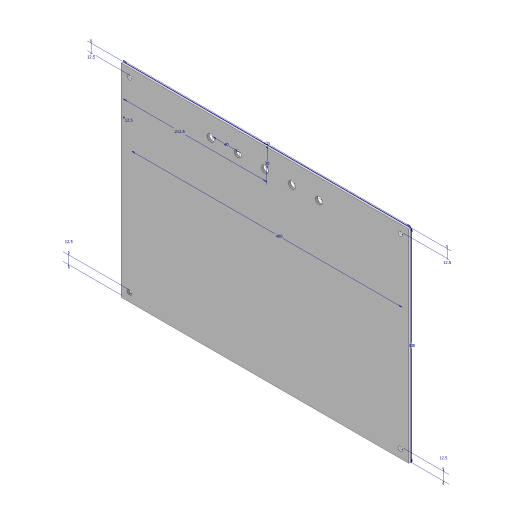
# Autodesk Inventor part: back_wall
Saved by Autodesk Inventor 2023 (Build 270158000, 158)
## iProperties
Created: 2024-06-07
Part Number: back_wall
Material: Generic
Document SubType Name: Modeling
Designer: nvladi
Density: 1 g/cm^3
Appearance: Default
Author: nvladi
Autodesk Inventor part; units mm, degrees
ref_plane "YZ Plane" through (0, 0, 0) normal (1, 0, 0) x (0, 1, 0)
ref_plane "XZ Plane" through (0, 0, 0) normal (0, 1, 0) x (-1, 0, 0)
ref_plane "XY Plane" through (0, 0, 0) normal (0, 0, 1) x (1, 0, 0)
sketch "Sketch1" plane through (0, 0, 0) normal (0, 0, 1) x (1, 0, 0)
  line L0 (0, 0) -> (425, 0)
  line L1 (425, 0) -> (425, 300)
  line L2 (425, 300) -> (0, 300)
  line L3 (0, 300) -> (0, 0)
  line L4 (12.5, 287.5) -> (12.5, 12.5) construction
  line L5 (412.5, 287.5) -> (412.5, 12.5) construction
  point P0 (132.5, 270)
  point P1 (172.5, 270)
  point P2 (212.5, 270)
  point P3 (252.5, 270)
  point P4 (292.5, 270)
  point P5 (212.5, 300)
  dimension "d0" = 425
  dimension "d1" = 300
  dimension "d2" = 400
  dimension "d3" = 12.5
  dimension "d4" = 12.5
  dimension "d5" = 12.5
  dimension "d6" = 12.5
  dimension "d7" = 12.5
  dimension "d19" = 40
  dimension "d24" = 212.5
  dimension "d32" = 30
  constraints: 12 end point, 4 coincident, 2 horizontal, 2 parallel, 2 perpendicular, 1 midpoint, 1 vertical, 4 other
  measures "d0" distance of L2.end L1.end
  measures "d1" distance of L1.end L0.end
  measures "d2" distance between parallel lines of L5 L4
  measures "d3" distance between parallel lines of L4 L3
  measures "d4" distance from line of point (12.5, 287.5) L2
  measures "d5" distance from line of L0 point (12.5, 12.5)
  measures "d6" distance from line of point (412.5, 287.5) L2
  measures "d7" distance from line of L0 point (412.5, 12.5)
  measures "d19" distance of point (132.5, 270) point (172.5, 270)
  measures "d24" distance from line of L3 point (212.5, 270)
  measures "d32" distance of point (212.5, 270) point (212.5, 300)
extrude "Extrusion1" add sketch "Sketch1" along normal blind 3
hole "Hole1" at (12.5, 287.5, 0) at (412.5, 287.5, 0) at (12.5, 12.5, 0) at (412.5, 12.5, 0) direction (0, 0, 1) diameter 6.4 end through all
hole "Hole2" at (132.5, 270, 0) at (172.5, 270, 0) at (212.5, 270, 0) at (252.5, 270, 0) at (292.5, 270, 0) direction (0, 0, 1) diameter 10 end through all
body "Solid1"
